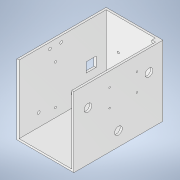
# Autodesk Inventor part: obudowa
Saved by Autodesk Inventor 2020 (Build 240168000, 168)
## iProperties
Created: 2020-08-28
Part Number: obudowa
Material: ABS Plastic
Document SubType Name: Modeling
Designer: Hesekiel
Density: 1.06 g/cm^3
Appearance: Smooth - White
Mass: 132.014 g
Surface Area: 857.121 cm^2
Volume: 124.542 cm^3
Sheet Metal Rule: Default
Author: Hesekiel
Autodesk Inventor part; units mm, degrees
ref_plane "YZ Plane" through (0, 0, 0) normal (1, 0, 0) x (0, 1, 0)
ref_plane "XZ Plane" through (0, 0, 0) normal (0, 1, 0) x (-1, 0, 0)
ref_plane "XY Plane" through (0, 0, 0) normal (0, 0, 1) x (1, 0, 0)
sketch "Sketch3" plane through (0, 0, 0) normal (0, 1, 0) x (-1, 0, 0)
  line L0 (-44, 50) -> (44, 50)
  line L1 (44, 50) -> (44, -50)
  line L2 (44, -50) -> (-44, -50)
  line L3 (-44, -50) -> (-44, 50)
  line L4 (-44, 50) -> (44, -50) construction
  line L5 (44, 50) -> (-44, -50) construction
  line L6 (44, 50) -> (-44, 50)
  line L7 (-44, 50) -> (-44, 47)
  line L8 (-44, 47) -> (44, 47)
  line L9 (44, 47) -> (44, 50)
  line L10 (44, 47) -> (41, 47)
  line L11 (41, 47) -> (41, -50)
  line L12 (41, -50) -> (44, -50)
  line L13 (44, -50) -> (44, 47)
  line L14 (-44, 47) -> (-41, 47)
  line L15 (-41, 47) -> (-41, -50)
  line L16 (-41, -50) -> (-44, -50)
  line L17 (-44, -50) -> (-44, 47)
  line L18 (41, -50) -> (-41, -50)
  line L19 (-41, -50) -> (-41, -47)
  line L20 (-41, -47) -> (41, -47)
  line L21 (41, -47) -> (41, -50)
  line L22 (41, 47) -> (34, 47)
  line L23 (34, 47) -> (34, -50)
  line L24 (34, -50) -> (37, -50)
  line L25 (37, -50) -> (37, 50)
  line L26 (34, 47) -> (34, 50)
  line L27 (41, 47) -> (41, 50)
  line L28 (-41, 47) -> (-41, 50)
  point P0 (0, 0)
  point P1 (37, -47)
  point P2 (37, 47)
  point P3 (34, -47)
  point P4 (37, 50)
  dimension "d33" = 88
  dimension "d34" = 100
  dimension "d35" = 88
  dimension "d36" = 3
  dimension "d37" = 3
  dimension "d38" = 3
  dimension "d39" = 3
  dimension "d63" = 7
  dimension "d64" = 3
  constraints: 58 end point, 11 point on line, 10 parallel, 7 perpendicular, 5 horizontal, 2 midpoint, 2 vertical
  measures "d33" distance of L1.end L2.end
  measures "d34" distance of L0.end L1.end
  measures "d35" distance of L8.end L7.end
  measures "d36" distance of L7.end L6.end
  measures "d37" distance of L12.end L11.end
  measures "d38" distance of L15.end L16.end
  measures "d39" distance of L18.end L19.end
  measures "d63" distance of L10.end L22.end
  measures "d64" distance of L23.end L24.end
extrude "Extrusion2" add sketch "Sketch3" along normal blind 100 contours L8 L15 L2 L3 | L8 L25 L20 L23 | L20 L23 L2 L15 | L20 L25 L2 L23
sketch "Sketch6" plane through (44, 0, -50) normal (0, 0, -1) x (-1, 0, 0)
  circle A0 centre (62.07, 7.54) radius 1.5875
  circle A1 centre (10, 12.62) radius 1.5875
  circle A2 centre (10, 40.56) radius 1.5875
  line L0 (7.46, 10.08) -> (7.46, 42.846)
  line L1 (7.46, 42.846) -> (10, 45.386)
  line L2 (10, 45.386) -> (10, 58.34)
  line L3 (10, 7.54) -> (7.46, 10.08)
  line L4 (10, 5) -> (10, 7.54)
  line L5 (76.04, 5) -> (10, 5)
  line L6 (76.04, 58.34) -> (76.04, 5)
  line L7 (10, 58.34) -> (76.04, 58.34)
  circle A3 centre (60.8, 55.8) radius 1.5875
  line L8 (0, 0) -> (81, 0) projected
  line L9 (0, 100) -> (81, 100) projected
  line L10 (0, 0) -> (0, 100) projected
  line L11 (0, 0) -> (0, 100) projected
  line L12 (0, 0) -> (10, 0)
  line L13 (78, 0) -> (3, 0) projected
  line L14 (10, 0) -> (10, 5)
  line L15 (81, 0) -> (81, 100) projected
  point P0 (44, 0)
  point P1 (85, 0)
  dimension "d52" = 10
  dimension "d53" = 5
  dimension "d54" = 90
  constraints: 20 end point, 4 centre point, 1 perpendicular, 1 point on line
  measures "d52" distance of L8.start L12.end
  measures "d53" distance of L12.end L14.end
  measures "d54" angle of L14 L12
extrude "Extrusion4" cut sketch "Sketch6" against normal up to surface (3 mm away) contours A0 | A1 | A2 | A3
sketch "Sketch9" plane through (-37, 0, -50) normal (-1, 0, 0) x (0, 0, 1)
  line L0 (17.33, 50.02) -> (31.33, 50.02) projected
  line L1 (31.33, 50.02) -> (31.33, 36.02) projected
  line L2 (31.33, 36.02) -> (17.33, 36.02) projected
  line L3 (17.33, 36.02) -> (17.33, 50.02) projected
  line L4 (17.65, 20.175) -> (32.65, 20.175) projected
  line L5 (32.65, 20.175) -> (32.65, 5.175) projected
  line L6 (32.65, 5.175) -> (17.65, 5.175) projected
  line L7 (17.65, 5.175) -> (17.65, 20.175) projected
  point P0 (50, 0)
extrude "Extrusion6" cut sketch "Sketch9" against normal up to surface (3 mm away)
sketch "Sketch10" plane through (44, 0, 50) normal (1, 0, 0) x (0, 0, -1)
  circle A0 centre (23.979, 79.591) radius 1.0922
  circle A1 centre (62.841, 79.591) radius 1.0922
  circle A2 centre (62.841, 54.191) radius 1.0922
  line L0 (21.82, 50) -> (21.82, 81.75)
  line L1 (65, 50) -> (21.82, 50)
  line L2 (65, 81.75) -> (65, 50)
  line L3 (21.82, 81.75) -> (65, 81.75)
  circle A3 centre (23.979, 54.191) radius 1.0922
  line L4 (3, 0) -> (100, 0) projected
  line L5 (100, 0) -> (100, 100) projected
  line L6 (3, 100) -> (100, 100) projected
  line L7 (100, 0) -> (100, 100) projected
  line L8 (100, 100) -> (65, 100)
  line L9 (3, 100) -> (100, 100) projected
  line L10 (100, 100) -> (135, 100) construction
  line L11 (100, 0) -> (100, 100) projected
  line L12 (65, 100) -> (65, 0)
  line L13 (100, 0) -> (3, 0) projected
  line L14 (3, 0) -> (3, 100) projected
  point P0 (50, 0)
  point P1 (0, 0)
  point P2 (0, 100)
  dimension "d67" = 35
  dimension "d68" = 180
  dimension "d75" = 100
  constraints: 14 end point, 4 centre point, 2 collinear, 1 horizontal, 1 point on line
  measures "d67" distance of L5.end L8.end
  measures "d68" angle of L8 L10
  measures "d75" distance of L8.end L12.end
extrude "Extrusion7" cut sketch "Sketch10" against normal up to surface (3 mm away) contours A0 | A1 | A2 | A3
sketch "Sketch11" plane through (-37, 0, -50) normal (-1, 0, 0) x (0, 0, 1)
  circle A0 centre (75.1, 71.8) radius 1.55
  circle A1 centre (75.1, 15.4) radius 1.55
  line L0 (67.45, 5) -> (82.75, 5)
  line L1 (67.45, 82.2) -> (82.75, 82.2)
  line L2 (95, 82.2) -> (95, 5)
  line L3 (55.2, 82.2) -> (55.2, 5)
  line L4 (32.65, 5.175) -> (17.65, 5.175) projected
  line L5 (17.65, 5.175) -> (17.65, 20.175) projected
  line L6 (17.65, 20.175) -> (32.65, 20.175) projected
  line L7 (32.65, 20.175) -> (32.65, 5.175) projected
  line L8 (31.33, 50.02) -> (31.33, 36.02) projected
  line L9 (31.33, 36.02) -> (17.33, 36.02) projected
  line L10 (17.33, 36.02) -> (17.33, 50.02) projected
  line L11 (17.33, 50.02) -> (31.33, 50.02) projected
  line L12 (0, 0) -> (97, 0) projected
  line L13 (0, 100) -> (97, 100) projected
  line L14 (0, 0) -> (0, 100) projected
  line L15 (100, 0) -> (100, 100) projected
  line L16 (100, 0) -> (100, 5)
  line L17 (100, 5) -> (95, 5)
  line L18 (97, 0) -> (97, 100) projected
  point P0 (50, 0)
  dimension "d71" = 5
  dimension "d72" = 5
  constraints: 12 end point, 2 centre point, 1 perpendicular, 1 point on line
  measures "d71" distance of L15.start L16.end
  measures "d72" distance of L16.end L17.end
extrude "Extrusion8" cut sketch "Sketch11" against normal up to surface (3 mm away) contours A0 | A1
sketch "Sketch12" plane through (-34, 0, -47) normal (0, 0, 1) x (1, 0, 0)
  circle A0 centre (17.2, 55.8) radius 1.5875 projected
  circle A1 centre (68, 40.56) radius 1.5875 projected
  circle A2 centre (15.93, 7.54) radius 1.5875 projected
  circle A3 centre (68, 12.62) radius 1.5875 projected
  line L0 (0, 0) -> (75, 0) projected
  line L1 (75, 0) -> (75, 100) projected
  line L2 (0, 100) -> (75, 100) projected
  line L3 (0, 0) -> (0, 100) projected
  line L4 (75, 0) -> (75, 100) projected
  line L5 (75, 100) -> (70, 100)
  line L6 (70, 100) -> (70, 70)
  line L7 (70, 70) -> (75, 70)
  line L8 (75, 70) -> (75, 100)
  point P0 (34, 0)
  dimension "d76" = 5
  dimension "d77" = 30
  constraints: 8 end point, 2 parallel, 1 horizontal, 1 perpendicular
  measures "d76" distance of L7.end L6.end
  measures "d77" distance of L6.end L5.end
extrude "Extrusion9" add sketch "Sketch12" along normal blind 2.4 contours L7 L6 L2 L1
sketch "Sketch13" plane through (-34, 0, -44.6) normal (0, 0, 1) x (1, 0, 0)
  line L0 (70, 100) -> (70, 70) projected
  line L1 (70, 70) -> (75, 70) projected
  line L2 (75, 100) -> (75, 70) projected
  line L3 (75, 100) -> (70, 100) projected
  line L4 (70, 100) -> (70, 70) projected
  line L5 (75, 100) -> (70, 100)
  line L6 (70, 100) -> (70, 97)
  line L7 (70, 97) -> (75, 97)
  line L8 (75, 97) -> (75, 100)
  point P0 (34, 0)
  dimension "d80" = 3
  constraints: 8 end point, 2 parallel, 1 horizontal, 1 perpendicular, 1 point on line
  measures "d80" distance of L6.end L5.end
extrude "Extrusion10" add sketch "Sketch13" along normal blind 2.4 contours L3 L2 L7 L0
sketch "Sketch14" plane through (-34, 0, -47) normal (0, 0, 1) x (1, 0, 0)
  line L0 (75, 0) -> (75, 70) projected
  line L1 (0, 0) -> (0, 100) projected
  line L2 (75, 0) -> (0, 0)
  line L3 (0, 0) -> (0, 3)
  line L4 (0, 3) -> (75, 3)
  line L5 (75, 3) -> (75, 0)
  point P0 (34, 0)
  dimension "d83" = 3
  constraints: 8 end point, 2 parallel, 1 horizontal, 1 perpendicular, 1 point on line
  measures "d83" distance of L2.end L3.end
extrude "Extrusion11" add sketch "Sketch14" along normal up to surface (94 mm away)
sketch "Sketch15" plane through (-37, 0, 47) normal (0, 0, 1) x (1, 0, 0)
  line L0 (0, 0) -> (81, 0) projected
  line L1 (81, 0) -> (81, 100) projected
  line L2 (78, 100) -> (81, 100) projected
  line L3 (78, 3) -> (78, 100) projected
  line L4 (3, 3) -> (78, 3) projected
  line L5 (3, 3) -> (3, 100) projected
  line L6 (0, 100) -> (3, 100) projected
  line L7 (0, 0) -> (0, 100) projected
  point P0 (37, 0)
extrude "Extrusion12" add sketch "Sketch15" along normal blind 30
sketch "Sketch16" plane through (-37, 0, -50) normal (-1, 0, 0) x (0, 0, 1)
  circle A0 centre (75.1, 15.4) radius 1.55 projected
  circle A1 centre (75.1, 71.8) radius 1.55 projected
  line L0 (17.65, 5.175) -> (17.65, 20.175) projected
  line L1 (17.65, 20.175) -> (32.65, 20.175) projected
  line L2 (32.65, 20.175) -> (32.65, 5.175) projected
  line L3 (32.65, 5.175) -> (17.65, 5.175) projected
  line L4 (17.33, 50.02) -> (31.33, 50.02) projected
  line L5 (31.33, 50.02) -> (31.33, 36.02) projected
  line L6 (31.33, 36.02) -> (17.33, 36.02) projected
  line L7 (17.33, 36.02) -> (17.33, 50.02) projected
  line L8 (0, 0) -> (127, 0) projected
  line L9 (127, 100) -> (127, 0) projected
  line L10 (0, 100) -> (127, 100) projected
  line L11 (0, 0) -> (0, 100) projected
  circle A2 centre (75.1, 71.8) radius 1.55 projected
  line L12 (75.1, 71.8) -> (75.1, 91.8)
  line L13 (75.1, 91.8) -> (83.1, 91.8)
  line L14 (75.1, 91.8) -> (67.1, 91.8)
  circle A3 centre (83.1, 91.8) radius 2
  circle A4 centre (67.1, 91.8) radius 2
  line L15 (127, 3) -> (127, 100) projected
  line L16 (127, 51.5) -> (71.1, 51.5)
  line L17 (75.1, 11.2) -> (83.1, 11.2)
  line L18 (75.1, 11.2) -> (67.1, 11.2)
  circle A5 centre (83.1, 11.2) radius 2
  circle A6 centre (67.1, 11.2) radius 2
  line L19 (83.1, 11.2) -> (91.1, 11.2)
  line L20 (67.1, 11.2) -> (59.1, 11.2)
  line L21 (127, 3) -> (3, 3) projected
  circle A7 centre (59.1, 11.2) radius 2
  circle A8 centre (91.1, 11.2) radius 2
  line L22 (91.1, 11.2) -> (99.1, 11.2)
  line L23 (99.1, 11.2) -> (99.1, 21.2)
  line L24 (99.1, 21.2) -> (51.1, 21.2)
  circle A9 centre (99.1, 21.2) radius 2
  circle A10 centre (51.1, 21.2) radius 2
  point P0 (50, 0)
  dimension "d88" = 20
  dimension "d89" = 8
  dimension "d90" = 8
  dimension "d91" = 4
  dimension "d92" = 4
  dimension "d95" = 8
  dimension "d96" = 8
  dimension "d97" = 4
  dimension "d98" = 4
  dimension "d99" = 8
  dimension "d100" = 10
  dimension "d101" = 48
  dimension "d102" = 4
  dimension "d103" = 4
  constraints: 22 end point, 8 centre point, 8 coincident, 5 symmetric about line, 4 horizontal, 2 perpendicular, 2 point on line, 1 midpoint, 1 parallel, 1 vertical, 2 other
  measures "d88" distance of L12.start L12.end
  measures "d89" distance of L12.end L13.end
  measures "d90" distance of L12.end L14.end
  measures "d91" diameter of A3
  measures "d92" diameter of A4
  measures "d95" distance of L19.start L19.end
  measures "d96" distance of L20.start L20.end
  measures "d97" diameter of A7
  measures "d98" diameter of A8
  measures "d99" distance of L22.start L22.end
  measures "d100" distance of L22.end L23.end
  measures "d101" distance of L23.end L24.end
  measures "d102" diameter of A9
  measures "d103" diameter of A10
extrude "Extrusion13" cut sketch "Sketch16" against normal up to surface (3 mm away) contours A3 | A4 | A9 L24 L23 | L23 L24 A9 | A10
sketch "Sketch17" plane through (44, 0, -50) normal (1, 0, 0) x (0, 0, -1)
  circle A0 centre (-37.159, 79.591) radius 1.0922 projected
  circle A1 centre (-76.021, 54.191) radius 1.0922 projected
  circle A2 centre (-37.159, 54.191) radius 1.0922 projected
  circle A3 centre (-76.021, 79.591) radius 1.0922 projected
  line L0 (0, 0) -> (-127, 0) projected
  line L1 (0, 0) -> (0, 100) projected
  line L2 (0, 100) -> (-127, 100) projected
  line L3 (-127, 0) -> (-127, 100) projected
  line L4 (-127, 0) -> (-127, 100) projected
  line L5 (-127, 50) -> (-107, 50)
  circle A4 centre (-107, 50) radius 5.5
  line L6 (0, 0) -> (-127, 0) projected
  line L7 (-63.5, 0) -> (-63.5, 20)
  circle A5 centre (-63.5, 20) radius 5.5
  line L8 (0, 0) -> (0, 100) projected
  line L9 (0, 50) -> (-20, 50.02)
  line L10 (-17.33, 50.02) -> (-31.33, 50.02) projected
  circle A6 centre (-20, 50.02) radius 5.5
  line L11 (-107, 50) -> (-107, 70)
  line L12 (-20, 50.02) -> (-20, 70.02)
  circle A7 centre (-107, 70) radius 5.5
  circle A8 centre (-20, 70.02) radius 5.5
  point P0 (-50, 0)
  dimension "d104" = 20
  dimension "d105" = 11
  dimension "d106" = 20
  dimension "d107" = 11
  dimension "d110" = 20
  dimension "d111" = 11
  dimension "d112" = 20
  dimension "d113" = 20
  dimension "d114" = 11
  dimension "d115" = 11
  constraints: 10 end point, 5 centre point, 5 coincident, 3 midpoint, 3 vertical, 1 horizontal, 1 point on line
  measures "d104" distance of L5.start L5.end
  measures "d105" diameter of A4
  measures "d106" distance of L7.start L7.end
  measures "d107" diameter of A5
  measures "d110" distance of L9.start L9.end
  measures "d111" diameter of A6
  measures "d112" distance of L11.start L11.end
  measures "d113" distance of L12.start L12.end
  measures "d114" diameter of A7
  measures "d115" diameter of A8
extrude "Extrusion14" cut sketch "Sketch17" against normal up to surface (3 mm away) contours A5 | A7 | A8
equation "\"BendRadius\" = Thickness"
equation "\"BendReliefWidth\" = Thickness"
equation "\"BendReliefDepth\" = 0.5 * Thickness"
equation "\"CornerReliefSize\" = 4 * Thickness"
equation "\"MinimumRemnant\" = 2 * Thickness"
equation "\"TransitionRadius\" = BendRadius"
equation "\"JacobiRadiusSize\" = Thickness"
equation "\"GapSize\" = Thickness"
equation "\"Thickness\" = 3"
body "Solid2"
